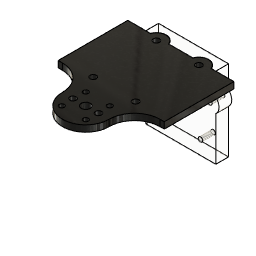
Top Plate Mosquito (Autodesk Fusion 360 design; units mm, degrees)
Autodesk Fusion 360 part; units mm, degrees
ref_plane "WorkPlane1" through (-5.7574, 23.4, 35) normal (0, 0, 1) x (1, 0, 0)
sketch "Sketch2" plane through (0, 24.7, 35) normal (0, 0, 1) x (1, 0, 0)
  arc A0 (-10.0949, 4.699) -> (-14.2426, 1.7) centre (-10, 0.2) ccw
  arc A1 (-5.7574, 1.7) -> (-9.9051, 4.699) centre (-10, 0.2) ccw
  arc A2 (-9.9051, 4.699) -> (-10.0949, 4.699) centre (-10, 0.2) ccw
  arc A3 (9.9051, 4.699) -> (5.7574, 1.7) centre (10, 0.2) ccw
  arc A4 (14.2426, 1.7) -> (10.0949, 4.699) centre (10, 0.2) ccw
  arc A5 (10.0949, 4.699) -> (9.9051, 4.699) centre (10, 0.2) ccw
  arc A6 (-9.9051, -34.099) -> (-5.7574, -31.1) centre (-10, -29.6) ccw
  arc A7 (-14.2426, -31.1) -> (-10.0949, -34.099) centre (-10, -29.6) ccw
  arc A8 (-10.0949, -34.099) -> (-9.9051, -34.099) centre (-10, -29.6) ccw
  arc A9 (10.0949, -34.099) -> (14.2426, -31.1) centre (10, -29.6) ccw
  arc A10 (5.7574, -31.1) -> (9.9051, -34.099) centre (10, -29.6) ccw
  arc A11 (9.9051, -34.099) -> (10.0949, -34.099) centre (10, -29.6) ccw
  circle A12 centre (-8, -22.2) radius 1.7 construction
  circle A13 centre (8, -7.2) radius 1.7 construction
  circle A14 centre (-8, -7.2) radius 1.7 construction
  circle A15 centre (8, -22.2) radius 1.7 construction
  line L0 (-25, 1.7) -> (-14.2426, 1.7)
  line L1 (-5.7574, 1.7) -> (5.7574, 1.7)
  line L2 (14.2426, 1.7) -> (25, 1.7)
  line L3 (25, 1.7) -> (25, -31.1)
  line L4 (-25, -31.1) -> (-25, 1.7)
  line L5 (25, -31.1) -> (14.2426, -31.1)
  line L6 (5.7574, -31.1) -> (-5.7574, -31.1)
  line L7 (-14.2426, -31.1) -> (-25, -31.1)
  circle A16 centre (10, 0.2) radius 1.465
  circle A17 centre (-10, 0.2) radius 1.465
  circle A18 centre (8, -22.2) radius 1.7 construction
  circle A19 centre (-8, -22.2) radius 1.7 construction
  line L8 (-14.2426, -31.1) -> (14.2426, -31.1) construction
  line L9 (14.2426, -31.1) -> (14.2426, -49.1) construction
  line L10 (14.2426, -49.1) -> (-14.2426, -49.1) construction
  line L11 (-14.2426, -49.1) -> (-14.2426, -31.1) construction
  circle A20 centre (0, -43.1) radius 2.1
  line L12 (0, -31.1) -> (0, -43.1) construction
  line L13 (-6, -43.1) -> (6, -43.1) construction
  circle A21 centre (10, -29.6) radius 1.465
  circle A22 centre (-10, -29.6) radius 1.465
  circle A23 centre (0, -43.1) radius 11
  line L14 (11, -43.1) -> (-11, -43.1) construction
  arc A24 (23, -31.1) -> (11, -43.1) centre (23, -43.1) ccw
  arc A25 (-11, -43.1) -> (-23, -31.1) centre (-23, -43.1) ccw
  dimension "d5282" = 18
  dimension "d5283" = 12
  dimension "d5288" = 12
  dimension "d6329" = 12
  dimension "d6330" = 4.2
  dimension "d6343" = 22
  constraint horizontal L8
  constraint vertical L9
  constraint horizontal L10
  constraint vertical L11
  constraint coincident A7.start L7.start
  constraint coincident A9.end L5.end
  constraint midpoint L6 L12.start
  constraint coincident A20.centre L12.end
  constraint horizontal L13
  constraint midpoint A20.centre L13
  constraint concentric A20 A23
  constraint coincident A23 L14.start
  constraint perpendicular L9 L14
  constraint midpoint A20.centre L14
  constraint tangent A23 A24
  constraint coincident L5 A24.start
  constraint tangent L5 A24
  constraint coincident L14 A24.end
  constraint vertical L12
  constraint symmetric L12 A24.start A25.end
  constraint symmetric L12 L14.start L14.end
  constraint symmetric L12 A24 A25
  measures "d5282" distance of A9.end L9.end
  measures "d5283" distance of L12.start A20.centre
  measures "d5288" distance of L13.start L13.end
  measures "d6329" distance of L12.start A20.centre
  measures "d6330" diameter of A20
  measures "d6343" diameter of A23
extrude "Extrude2" add sketch "Sketch2" along normal blind 3 makes body 1
hole "Hole1" at (-6, -18.4, 35) at (6, -18.4, 35) direction (0, 0, 1) diameter 2.9 depth 10 tip angle 180 bodies 1
sketch "Sketch10" plane through (0, 0, 38) normal (0, 0, 1) x (-1, 0, 0)
  circle A0 centre (6, 18.4) radius 1.45
  circle A1 centre (-6, 18.4) radius 1.45
  arc A2 (11, 18.4) -> (-11, 18.4) centre (0, 18.4) ccw
  line L0 (-23, 6.4) -> (-25, 6.4)
  line L1 (-25, 6.4) -> (-25, -26.4)
  line L2 (-25, -26.4) -> (-14.2426, -26.4)
  arc A3 (-14.2426, -26.4) -> (-5.7574, -26.4) centre (-10, -24.9) ccw
  line L3 (-5.7574, -26.4) -> (5.7574, -26.4)
  arc A4 (5.7574, -26.4) -> (14.2426, -26.4) centre (10, -24.9) ccw
  line L4 (14.2426, -26.4) -> (25, -26.4)
  line L5 (25, -26.4) -> (25, 6.4)
  line L6 (25, 6.4) -> (23, 6.4)
  circle A5 centre (-10, 4.9) radius 1.465
  circle A6 centre (0, 18.4) radius 2.1
  circle A7 centre (10, -24.9) radius 1.465
  circle A8 centre (-10, -24.9) radius 1.465
  circle A9 centre (10, 4.9) radius 1.465
  circle A10 centre (0, 18.4) radius 2.1
  circle A11 centre (0, 18.4) radius 11
  line L7 (-5.657, 24.057) -> (5.657, 24.057) construction
  line L8 (5.657, 24.057) -> (5.657, 12.743) construction
  line L9 (5.657, 12.743) -> (-5.657, 12.743) construction
  line L10 (-5.657, 12.743) -> (-5.657, 24.057) construction
  line L11 (-5.657, 24.057) -> (5.657, 12.743) construction
  line L12 (5.657, 24.057) -> (-5.657, 12.743) construction
  arc A12 (11, 18.4) -> (23, 6.4) centre (23, 18.4) ccw
  arc A13 (-23, 6.4) -> (-11, 18.4) centre (-23, 18.4) ccw
  point P0 (0, 18.4)
  dimension "d6344" = 11.314
  dimension "d6345" = 11.314
  constraint concentric A10 A11
  constraint equal A2 A11
  constraint horizontal L7
  constraint perpendicular L7 L8
  constraint parallel L7 L9
  constraint parallel L8 L10
  constraint coincident L11 P0
  constraint coincident L12 P0
  constraint coincident P0 A2.centre
  measures "d6344" distance of L8.end L9.end
  measures "d6345" distance of L7.end L8.end
hole "Hole5" at (5.657, -12.743, 38) at (-5.657, -12.743, 38) at (-5.657, -24.057, 38) at (5.657, -24.057, 38) direction (0, 0, -1) diameter 2.4 end up to surface (3 mm away) bodies 1
sketch "Sketch3" plane through (0, 0, 38) normal (0, 0, 1) x (-1, 0, 0)
  circle A0 centre (6, 18.4) radius 1.45
  circle A1 centre (-6, 18.4) radius 1.45
  line L0 (-23, 6.4) -> (-25, 6.4)
  line L1 (-25, 6.4) -> (-25, -26.4)
  line L2 (-25, -26.4) -> (-14.2426, -26.4)
  arc A2 (-14.2426, -26.4) -> (-5.7574, -26.4) centre (-10, -24.9) ccw
  line L3 (-5.7574, -26.4) -> (5.7574, -26.4)
  arc A3 (5.7574, -26.4) -> (14.2426, -26.4) centre (10, -24.9) ccw
  line L4 (14.2426, -26.4) -> (25, -26.4)
  line L5 (25, -26.4) -> (25, 6.4)
  line L6 (25, 6.4) -> (23, 6.4)
  circle A4 centre (10, -24.9) radius 1.465
  circle A5 centre (0, 18.4) radius 2.1
  circle A6 centre (-10, 4.9) radius 1.465
  circle A7 centre (10, 4.9) radius 1.465
  circle A8 centre (-10, -24.9) radius 1.465
  line L7 (16.5, -26.4) -> (-16.5, -26.4)
  line L8 (-16.5, -26.4) -> (-16.5, -32.4)
  line L9 (-16.5, -32.4) -> (16.5, -32.4)
  line L10 (16.5, -32.4) -> (16.5, -26.4)
  line L11 (0, -26.4) -> (0, -32.4) construction
  arc A9 (11, 18.4) -> (-11, 18.4) centre (0, 18.4) ccw
  arc A10 (11, 18.4) -> (23, 6.4) centre (23, 18.4) ccw
  arc A11 (-23, 6.4) -> (-11, 18.4) centre (-23, 18.4) ccw
  circle A12 centre (5.657, 24.057) radius 1.2
  circle A13 centre (-5.657, 12.743) radius 1.2
  circle A14 centre (5.657, 12.743) radius 1.2
  circle A15 centre (-5.657, 24.057) radius 1.2
  dimension "d5823" = 33
  dimension "d5826" = 3
  constraint horizontal L7
  constraint vertical L8
  constraint horizontal L9
  constraint vertical L10
  constraint midpoint L3 L11.start
  constraint perpendicular L3 L11
  constraint midpoint L9 L11.end
  constraint coincident L2 L7.end
  measures "d5823" distance of L7.start L7.end
  measures "d5826" distance of A2 L9
extrude "Extrude3" add sketch "Sketch3" against normal up to surface (38 mm away) separate body contours L2 A2 L3 A3 L4 L7 L8 L9 L10 makes body 2
move_face "OffsetFaces1" offset -0.1 2 faces at (5.9217, 26.802, 25.3333) (-14.0783, 26.802, 25.3333) on bodies 2
sketch "Sketch8" plane through (0, 0, 0) normal (0, 0, -1) x (1, 0, 0)
  line L0 (16.5, -26.4) -> (14.3486, -26.4)
  arc A0 (5.6514, -26.4) -> (14.3486, -26.4) centre (10, -24.9) ccw
  line L1 (5.6514, -26.4) -> (-5.6514, -26.4)
  arc A1 (-14.3486, -26.4) -> (-5.6514, -26.4) centre (-10, -24.9) ccw
  line L2 (-14.3486, -26.4) -> (-16.5, -26.4)
  line L3 (-16.5, -26.4) -> (-16.5, -32.4)
  line L4 (-16.5, -32.4) -> (16.5, -32.4)
  line L5 (16.5, -32.4) -> (16.5, -26.4)
  line L6 (-16.5, -26.4) -> (16.5, -26.4)
  constraint coincident L2.end L3.start
  constraint coincident L0.start L5.end
extrude "Extrude5" add sketch "Sketch8" against normal blind 24.5 contours A0 L6 | A1 L6 bodies 2 1
sketch "Sketch7" plane through (0, 32.4, 0) normal (0, 1, 0) x (-1, 0, 0)
  line L0 (16.5, 38) -> (-16.5, 38)
  line L1 (-16.5, 38) -> (-16.5, 0)
  line L2 (-16.5, 0) -> (16.5, 0)
  line L3 (16.5, 0) -> (16.5, 38)
  line L4 (0, 38) -> (0, 24) construction
  line L5 (0, 24) -> (13.5, 24) construction
  point P0 (-13.5, 24)
  dimension "d5830" = 13.5
  dimension "d5831" = 24
  constraint midpoint L0 L4.start
  constraint perpendicular L0 L4
  constraint perpendicular L3 L5
  constraint symmetric L4 L5.end P0
  measures "d5830" distance of L4.end L5.end
  measures "d5831" distance of L2 L5
hole "Hole3" at (-13.5, 32.4, 24) at (13.5, 32.4, 24) direction (0, -1, 0) diameter 2.529 depth 15 tip angle 118 bodies 1 2
thread "Thread1" "ISO Metric profile 3.0 M3x0.5 6H"
sketch "Sketch9" plane through (0, 32.4, 0) normal (0, 1, 0) x (-1, 0, 0)
  line L0 (16.5, 0) -> (16.5, 38)
  line L1 (16.5, 38) -> (-16.5, 38)
  line L2 (-16.5, 38) -> (-16.5, 0)
  line L3 (-16.5, 0) -> (16.5, 0)
  circle A0 centre (13.5, 24) radius 1.2645
  circle A1 centre (-13.5, 24) radius 1.2645
  circle A2 centre (13.5, 24) radius 4.5
  circle A3 centre (-13.5, 24) radius 4.5
  line L4 (0, 0) -> (0, 6.5) construction
  line L5 (0, 6.5) -> (9.25, 6.5) construction
  point P0 (-9.25, 6.5)
  dimension "d5839" = 9
  dimension "d5846" = 9.25
  dimension "d5847" = 6.5
  constraint concentric A0 A2
  constraint concentric A1 A3
  constraint equal A2 A3
  constraint midpoint L3 L4.start
  constraint perpendicular L3 L4
  constraint perpendicular L0 L5
  constraint symmetric L4 L5.end P0
  measures "d5839" diameter of A2
  measures "d5846" distance of L4.end L5.end
  measures "d5847" distance of L4.start L4.end
hole "Hole4" at (9.25, 32.4, 6.5) at (-9.25, 32.4, 6.5) direction (0, -1, 0) diameter 2.076 end up to surface (9 mm away) bodies 1 2
thread "Thread2" "ISO Metric profile 2.5 M2.5x0.45 6H"
extrude "Extrude6" add sketch "Sketch9" against normal up to surface (6 mm away) contours L0 A2 | L2 A3 picked at (16.9853, 24.2096) picked at (-17.2342, 23.585) bodies 1 2
equation "d5282 = d6329 + 6 mm"
equation "d5830 = ( 27 / 2 ) * 1 mm"
equation "d6345 = d6344"
named bodies: "Top Plate Mosquito"
